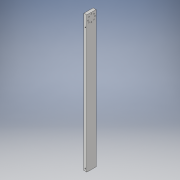
# Autodesk Inventor part: GlyphPlateLeftSide
Saved by Autodesk Inventor 2017 (Build 210142000, 142)
## iProperties
Created: 2018-01-27
Part Number: GlyphPlateLeftSide
Material: Generic
Document SubType Name: Modeling
Designer: User
Density: 1 g/cm^3
Appearance: Default
Author: User
Autodesk Inventor part; units mm, degrees
ref_plane "YZ Plane" through (0, 0, 0) normal (1, 0, 0) x (0, 1, 0)
ref_plane "XZ Plane" through (0, 0, 0) normal (0, 1, 0) x (-1, 0, 0)
ref_plane "XY Plane" through (0, 0, 0) normal (0, 0, 1) x (1, 0, 0)
sketch "Sketch1" plane through (0, 0, 0) normal (0, 0, 1) x (1, 0, 0)
  line L0 (0, 0) -> (8.0518, 0)
  line L1 (8.0518, 0) -> (8.0518, 374.65)
  line L2 (8.0518, 374.65) -> (0, 374.65)
  line L3 (0, 374.65) -> (0, 0)
  dimension "d0" = 8.0518
  dimension "d1" = 374.65
  constraints: 8 end point, 2 parallel, 1 horizontal, 1 perpendicular
  measures "d0" distance of L2.end L1.end
  measures "d1" distance of L1.end L0.end
extrude "Extrusion1" add sketch "Sketch1" along normal blind 25.4
sketch "Sketch2" plane through (0, 0, 25.4) normal (0, 0, 1) x (1, 0, 0)
  line L0 (0, 0) -> (8.0518, 0) projected
  line L1 (4.0259, 0) -> (4.0259, 6.35)
  circle A0 centre (4.0259, 6.35) radius 1.778
  line L2 (8.0518, 374.65) -> (0, 374.65) projected
  line L3 (4.0259, 374.65) -> (4.0259, 342.9)
  circle A1 centre (4.0259, 342.9) radius 1.778
  dimension "d4" = 6.35
  dimension "d5" = 3.556
  dimension "d6" = 31.75
  dimension "d7" = 3.556
  constraints: 4 coincident, 4 end point, 2 centre point, 2 midpoint, 2 vertical
  measures "d4" distance of L1.start L1.end
  measures "d5" diameter of A0
  measures "d6" distance of L3.start L3.end
  measures "d7" diameter of A1
hole "Hole1" at (4.0259, 342.9, 25.4) at (4.0259, 6.35, 25.4) direction (0, 0, -1) diameter 2.6416 depth 25.4 tip angle 118 thread size "6-32 UNC" class "2B" standard "ANSI Unified Screw Threads"
sketch "Sketch3" plane through (8.0518, 0, 0) normal (1, 0, 0) x (0, 0, -1)
  line L0 (0, 374.65) -> (-25.4, 374.65) projected
  circle A0 centre (-12.7, 360.68) radius 9.779
  point P0 (0, 0)
  point P1 (-21.59, 359.41)
  point P2 (-12.7, 370.459)
  point P3 (-19.6148, 367.5948)
  point P4 (-22.479, 360.68)
  point P5 (-19.6148, 353.7652)
  point P6 (-12.7, 350.901)
  point P7 (-5.7852, 353.7652)
  point P8 (-2.921, 360.68)
  point P9 (-5.7852, 367.5948)
  dimension "d36" = 19.558
  dimension "d35" = 13.97
  dimension "d39" = 360
  constraints: 1 vertical alignment, 11 other
  measures "d35" distance from line of L0 point (-12.7, 360.68)
hole "Hole2" at (8.0518, 359.41, 21.59) at (8.0518, 367.5948, 19.6148) at (8.0518, 370.459, 12.7) at (8.0518, 367.5948, 5.7852) at (8.0518, 360.68, 2.921) at (8.0518, 353.7652, 5.7852) at (8.0518, 350.901, 12.7) at (8.0518, 353.7652, 19.6148) direction (-1, 0, 0) diameter 2.7178 depth 25.4 tip angle 118
body "Solid1"
